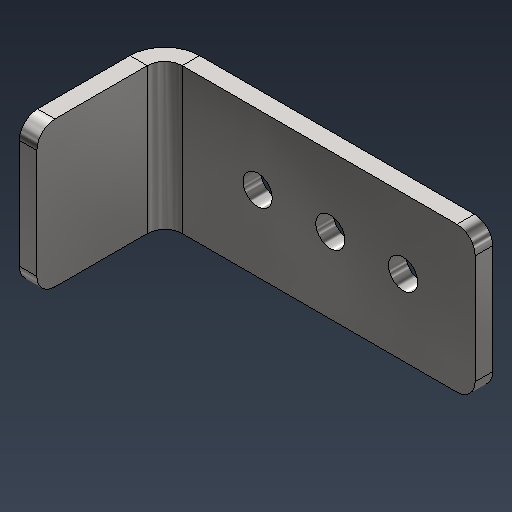
# Autodesk Inventor part: MOUNT,FLANGE,BELLYPAN
Saved by Autodesk Inventor 2026 (Build 300175050, 175E)
## iProperties
Created: 2026-02-21
Part Number: MOUNT,FLANGE,BELLYPAN
Material: Steel, Alloy
Document SubType Name: Sheet Metal
Designer: Jthib
Mass: 44.8288 g
Surface Area: 45.6367 cm^2
Volume: 5.79933 cm^3
Density: 7.73 g/cm^3
Sheet Metal Rule: Default
Appearance: Semi-Polished
Author: Jthib
Autodesk Inventor part; units mm, degrees
ref_plane "YZ Plane" through (0, 0, 0) normal (1, 0, 0) x (0, 1, 0)
ref_plane "XZ Plane" through (0, 0, 0) normal (0, 1, 0) x (-1, 0, 0)
ref_plane "XY Plane" through (0, 0, 0) normal (0, 0, 1) x (1, 0, 0)
sketch "Sketch1" plane through (0, 0, 0) normal (0, 0, 1) x (1, 0, 0)
  line L0 (25.4, 12.7) -> (-25.4, 12.7)
  line L1 (-25.4, 12.7) -> (-25.4, -12.7) construction
  line L2 (-25.4, -12.7) -> (25.4, -12.7)
  line L3 (25.4, -12.7) -> (25.4, 12.7)
  line L4 (25.4, 12.7) -> (-25.4, -12.7) construction
  line L5 (-25.4, 12.7) -> (25.4, -12.7) construction
  line L6 (-25.4, -12.7) -> (-28.829, -12.7)
  line L7 (-28.829, -12.7) -> (-28.829, 12.7)
  line L8 (-28.829, 12.7) -> (-25.4, 12.7)
  point P0 (0, 0)
  dimension "d0" = 25.4
  dimension "d1" = 50.8
  dimension "d2" = 3.429
  measures "d0" distance of L0.end L1.end
  measures "d1" distance of L0.start L0.end
  measures "d2" distance of L1.end L6.end
extrude "Plate1" add sketch "Sketch1" along normal blind 3.048
sketch "Sketch2" plane through (-28.829, -12.7, 3.048) normal (-1, 0, 0) x (0, -1, 0)
  line L0 (-25.4, 0) -> (0, 0)
  line L1 (0, 0) -> (0, 22.352)
  line L2 (0, 22.352) -> (-25.4, 22.352)
  line L3 (-25.4, 22.352) -> (-25.4, 0)
  constraints: 6 end point, 1 horizontal, 1 perpendicular, 1 vertical
edge flange "Flange1" height 25.4 angle 90 thickness 3.048 bend radius 3.048 thickness toward (-1, 0, 0) relief tear relief width 3.048 relief depth 1.524 edges at (-28.829, 0, 3.048) wall of the first edge with corners at (-28.829, 12.7, 3.048) (-28.829, -12.7, 3.048) (-28.829, -12.7, 25.4) (-28.829, 12.7, 25.4)
bend "Bend1"
corner "Corner1"
sketch "Sketch3" plane through (0, 0, 3.048) normal (0, 0, 1) x (1, 0, 0)
  point P0 (0, 0)
  point P1 (0.0945, 0.5029)
hole "Hole1" at (0.0945, 0.5029, 3.048) direction (0, 0, -1) diameter 5.1054 end through all clearance for "Flat Head Machine Screw (82)" size "#10" standard "Ansi Unified Screw Threads"
pattern_linear "Rectangular Pattern1" count 3 spacing 12.7 along (1, 0, 0) of "Hole1" first direction both ways yes
fillet "Corner Round1" radius 3.175 4 edges at (25.4, -12.7, 1.524) (25.4, 12.7, 1.524) (-30.353, 12.7, 25.4) (-30.353, -12.7, 25.4)
equation "\"d19\" = Thickness"
equation "\"d3\" = Thickness"
equation "\"d4\" = BendReliefWidth"
equation "\"d5\" = BendReliefDepth"
equation "\"d6\" = MinimumRemnant"
equation "\"d7\" = TransitionRadius"
equation "\"d10\" = BendRadius"
equation "\"d11\" = CornerReliefSize"
equation "\"d12\" = GapSize"
equation "\"d13\" = JacobiRadiusSize"
equation "\"BendRadius\" = Thickness"
equation "\"BendReliefWidth\" = Thickness"
equation "\"BendReliefDepth\" = 0.5 * Thickness"
equation "\"CornerReliefSize\" = 4 * Thickness"
equation "\"MinimumRemnant\" = 2 * Thickness"
equation "\"TransitionRadius\" = BendRadius"
equation "\"JacobiRadiusSize\" = BendRadius"
equation "\"GapSize\" = Thickness"
equation "\"Thickness\" = 3.048"
body "Solid1"
